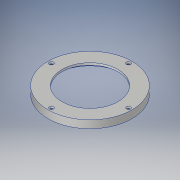
# Autodesk Inventor part: sensor2_lock
Saved by Autodesk Inventor 2018 (Build 220112000, 112)
## iProperties
Created: 2021-04-25
Part Number: sensor2_lock
Material: Aluminum 6061
Document SubType Name: Modeling
Designer: Ramana Bharathi
Density: 2.7 g/cm^3
Appearance: Aluminum - Flat
Mass: 124.546 g
Surface Area: 203.173 cm^2
Volume: 46.128 cm^3
Author: Ramana Bharathi
Autodesk Inventor part; units mm, degrees
ref_plane "YZ Plane" through (0, 0, 0) normal (1, 0, 0) x (0, 1, 0)
ref_plane "XZ Plane" through (0, 0, 0) normal (0, 1, 0) x (-1, 0, 0)
ref_plane "XY Plane" through (0, 0, 0) normal (0, 0, 1) x (1, 0, 0)
sketch "Sketch1" plane through (0, 0, 0) normal (0, 1, 0) x (-1, 0, 0)
  circle A0 centre (0, 0) radius 60
  dimension "d0" = 120
  constraints: 1 centre point, 1 coincident
  measures "d0" diameter of A0
extrude "Extrusion1" add sketch "Sketch1" along normal blind 11
sketch "Sketch3" plane through (0, 11, 0) normal (0, 1, 0) x (1, 0, 0)
  circle A0 centre (0, 0) radius 40
  dimension "d6" = 80
  constraints: 1 centre point, 1 coincident
  measures "d6" diameter of A0
extrude "Extrusion3" cut sketch "Sketch3" against normal through all
sketch "Sketch2" plane through (0, 0, 0) normal (0, -1, 0) x (1, 0, 0)
  circle A0 centre (0, 0) radius 50
  dimension "d3" = 100
  constraints: 1 centre point, 1 coincident
  measures "d3" diameter of A0
extrude "Extrusion2" cut sketch "Sketch2" against normal blind 8
sketch "Sketch4" plane through (0, 11, 0) normal (0, 1, 0) x (1, 0, 0)
  circle A0 centre (0, 0) radius 55
  circle A1 centre (0, 55) radius 1.5
  circle A2 centre (-55, 0) radius 1.5
  circle A3 centre (0, -55) radius 1.5
  circle A4 centre (55, 0) radius 1.5
  dimension "d9" = 110
  dimension "d10" = 3
  dimension "d13" = 360
  constraints: 4 centre point, 1 coincident, 1 vertical alignment, 11 other
  measures "d10" diameter of A1
hole "Hole1" at (0, 11, -55) at (-55, 11, 0) at (0, 11, 55) at (55, 11, 0) direction (0, -1, 0) diameter 3 end through all countersink diameter 6 countersink angle 90
thread "Thread1" size "M3x0.5" class "6H" standard "ANSI Metric M Profile" full length
thread "Thread2" size "M3x0.5" class "6H" standard "ANSI Metric M Profile" full length
thread "Thread3" size "M3x0.5" class "6H" standard "ANSI Metric M Profile" full length
thread "Thread4" size "M3x0.5" class "6H" standard "ANSI Metric M Profile" full length
body "Solid1"
